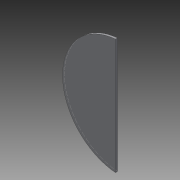
# Autodesk Inventor part: Mid Plate
Saved by Autodesk Inventor 2015 (Build 190159000, 159)
## iProperties
Created: 2014-08-15
Part Number: Mid Plate
Material: Generic
Document SubType Name: Modeling
Designer: karl
Density: 1 g/cm^3
Appearance: Default
Author: karl
Autodesk Inventor part; units mm, degrees
ref_plane "YZ Plane" through (0, 0, 0) normal (1, 0, 0) x (0, 1, 0)
ref_plane "XZ Plane" through (0, 0, 0) normal (0, 1, 0) x (-1, 0, 0)
ref_plane "XY Plane" through (0, 0, 0) normal (0, 0, 1) x (1, 0, 0)
sketch "Sketch1" plane through (0, 0, 0) normal (0, 1, 0) x (-1, 0, 0)
  circle A0 centre (0, 0) radius 85
  line L0 (7.5, 84.6685) -> (7.5, -84.6685)
  dimension "d0" = 170
  dimension "d1" = 7.5
  constraints: 2 end point, 2 point on circle, 1 centre point, 1 coincident, 1 vertical
  measures "d0" diameter of A0
  measures "d1" distance from line of point (0, 0) L0
extrude "Extrusion1" add sketch "Sketch1" along normal blind 3 contours A0 L0 picked at (34.1822, 19.1304)
sketch "Sketch2" plane through (0, 3, 0) normal (0, 1, 0) x (1, 0, 0)
  line L0 (-20, 55) -> (-58, 55) construction
  line L1 (-58, 55) -> (-58, -55) construction
  line L2 (-58, -55) -> (-20, -55) construction
  line L3 (-20, -55) -> (-20, 55) construction
  line L4 (-20, 40) -> (-17, 40)
  line L5 (-17, 40) -> (-17, 20)
  line L6 (-17, 20) -> (-20, 20)
  line L7 (-20, 20) -> (-20, 40)
  line L8 (-20, 55) -> (-58, 55)
  line L9 (-58, 55) -> (-58, -55)
  line L10 (-58, -55) -> (-20, -55)
  line L11 (-20, -55) -> (-20, 55)
  line L12 (-20, -20) -> (-17, -20)
  line L13 (-17, -20) -> (-17, -40)
  line L14 (-17, -40) -> (-20, -40)
  line L15 (-20, -40) -> (-20, -20)
  line L16 (-58, 40) -> (-61, 40)
  line L17 (-61, 40) -> (-61, 20)
  line L18 (-61, 20) -> (-58, 20)
  line L19 (-58, 20) -> (-58, 40)
  line L20 (-58, -20) -> (-61, -20)
  line L21 (-61, -20) -> (-61, -40)
  line L22 (-61, -40) -> (-58, -40)
  line L23 (-58, -40) -> (-58, -20)
  line L24 (-34, 55) -> (-44, 55)
  line L25 (-44, 55) -> (-44, 58)
  line L26 (-44, 58) -> (-34, 58)
  line L27 (-34, 58) -> (-34, 55)
  line L28 (-34, -55) -> (-44, -55)
  line L29 (-44, -55) -> (-44, -58)
  line L30 (-44, -58) -> (-34, -58)
  line L31 (-34, -58) -> (-34, -55)
  point P0 (0, 0)
  point P1 (-20, 0)
  point P2 (-39, 58)
  point P3 (-39, 55)
  dimension "d4" = 38
  dimension "d5" = 110
  dimension "d6" = 20
  dimension "d7" = 3
  dimension "d8" = 20
  dimension "d9" = 20
  dimension "d10" = 3
  dimension "d11" = 20
  dimension "d12" = 20
  dimension "d13" = 3
  dimension "d14" = 10
  dimension "d15" = 3
  dimension "d16" = 10
  dimension "d17" = 3
  constraints: 64 end point, 16 parallel, 8 horizontal, 8 perpendicular, 8 point on line, 4 collinear, 3 midpoint, 1 horizontal alignment, 1 vertical alignment
  measures "d4" distance of L2.end L1.end
  measures "d5" distance of L1.end L0.end
  measures "d6" distance from line of point (0, 0) L3
  measures "d7" distance of L5.end L6.end
  measures "d8" distance of L4.end L5.end
  measures "d9" distance from line of point (0, 0) L6
  measures "d10" distance of L13.end L14.end
  measures "d11" distance of L12.end L13.end
  measures "d12" distance from line of point (0, 0) L12
  measures "d13" distance between parallel lines of L1 L17
  measures "d14" distance of L25.end L26.end
  measures "d15" distance of L24.end L25.end
  measures "d16" distance of L30.end L29.end
  measures "d17" distance of L29.end L28.end
extrude "Extrusion2" cut sketch "Sketch2" against normal blind 3
sketch "Sketch3" plane through (0, 3, 0) normal (0, 1, 0) x (1, 0, 0)
  line L0 (-66, 1.5) -> (-76, 1.5)
  line L1 (-76, 1.5) -> (-76, -1.5)
  line L2 (-76, -1.5) -> (-66, -1.5)
  line L3 (-66, -1.5) -> (-66, 1.5)
  line L4 (-61, 20) -> (-61, 40) projected
  line L5 (-58, -20) -> (-58, 20) projected
  point P0 (0, 0)
  point P1 (-66, 0)
  point P2 (-58, 0)
  dimension "d20" = 10
  dimension "d21" = 3
  dimension "d22" = 5
  constraints: 8 end point, 2 midpoint, 2 parallel, 1 horizontal, 1 horizontal alignment, 1 perpendicular
  measures "d20" distance of L2.end L1.end
  measures "d21" distance of L1.end L0.end
  measures "d22" distance between parallel lines of L3 L4
extrude "Extrusion3" cut sketch "Sketch3" against normal blind 3
sketch "Sketch4" plane through (0, 3, 0) normal (0, 1, 0) x (1, 0, 0)
  line L0 (-7.5, -84.6685) -> (-7.5, 84.6685) projected
  line L1 (-7.5, 75) -> (-25, 75)
  line L2 (-25, 75) -> (-25, 60)
  line L3 (-25, 60) -> (-7.5, 60)
  line L4 (-7.5, 60) -> (-7.5, 75)
  point P0 (0, 0)
  dimension "d25" = 25
  dimension "d26" = 60
  dimension "d27" = 15
  constraints: 8 end point, 2 parallel, 1 horizontal, 1 perpendicular, 1 point on line
  measures "d25" distance from line of L2 point (0, 0)
  measures "d26" distance from line of point (0, 0) L3
  measures "d27" distance between parallel lines of L3 L1
extrude "Extrusion4" cut sketch "Sketch4" against normal blind 3
mirror "Mirror1" about plane through (0, 0, 0) normal (0, 0, 1) of "Extrusion4"
sketch "Sketch5" plane through (0, 3, 0) normal (0, 1, 0) x (1, 0, 0)
  point P0 (0, 0)
equation "\"d12\" = d9"
body "Solid1"
